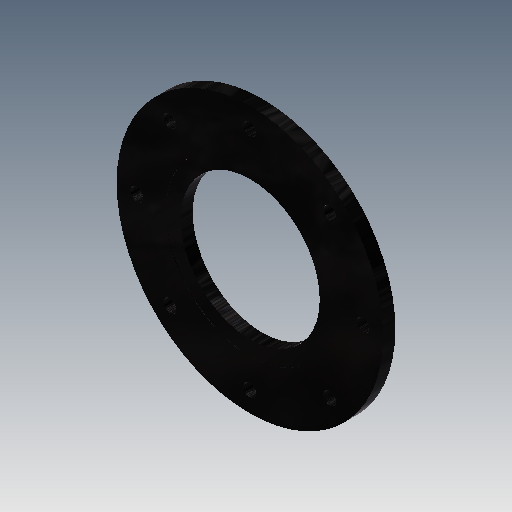
# Autodesk Inventor part: 軸受けワッシャB_ダブルスラスト用(厚さ2mm_ポケットあり_ジュラコン)
Saved by Autodesk Inventor 2019.4 (Build 234330000, 330)
## iProperties
Created: 2018-08-09
Part Number: 軸受けワッシャB_ダブルスラスト用(厚さ2mm_ポケットあり_ジュラコン)
Material: アセタール樹脂、黒
Document SubType Name: Modeling
Designer: Owner
Mass: 9.99263 g
Surface Area: 58.7838 cm^2
Volume: 7.01237 cm^3
Density: 1.425 g/cm^3
Appearance: 滑らか - 黒
Author: Owner
Autodesk Inventor part; units mm, degrees
ref_plane "YZ Plane" through (0, 0, 0) normal (1, 0, 0) x (0, 1, 0)
ref_plane "XZ Plane" through (0, 0, 0) normal (0, 1, 0) x (-1, 0, 0)
ref_plane "XY Plane" through (0, 0, 0) normal (0, 0, 1) x (1, 0, 0)
sketch "スケッチ1" plane through (0, 0, 0) normal (0, 0, 1) x (1, 0, 0)
  circle A0 centre (0, 0) radius 16.75 construction
  circle A1 centre (0, 0) radius 32.5
  circle A2 centre (0, 0) radius 27.6 construction
  circle A3 centre (27.6, 0) radius 1.6
  circle A4 centre (19.5161, 19.5161) radius 1.6
  circle A5 centre (0, 27.6) radius 1.6
  circle A6 centre (-19.5161, 19.5161) radius 1.6
  circle A7 centre (-27.6, 0) radius 1.6
  circle A8 centre (-19.5161, -19.5161) radius 1.6
  circle A9 centre (0, -27.6) radius 1.6
  circle A10 centre (19.5161, -19.5161) radius 1.6
  circle A11 centre (0, 0) radius 16.95
  dimension "d11" = 55.2
  dimension "d9" = 65
  dimension "d10" = 33.5
  dimension "d12" = 3.2
  dimension "d15" = 360
  dimension "d17" = 33.9
  constraints: 11 centre point, 1 coincident, 1 horizontal alignment, 19 other
  measures "d9" diameter of A1
  measures "d10" diameter of A0
  measures "d12" diameter of A3
  measures "d17" diameter of A11
extrude "押し出し3" add sketch "スケッチ1" along normal blind 3
sketch "スケッチ3" plane through (0, 0, 3) normal (0, 0, 1) x (1, 0, 0)
  circle A0 centre (0, 0) radius 32.5 projected
  circle A1 centre (0, 0) radius 20.5 projected
  circle A2 centre (0, 0) radius 16.95 projected
  circle A3 centre (0, 0) radius 20.5
  circle A4 centre (0, 0) radius 16.95
  constraints: 2 centre point, 2 coincident, 1 concentric
extrude "押し出し4" cut sketch "スケッチ3" against normal blind 0.1 contours A1
